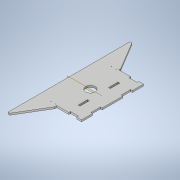
# Autodesk Inventor part: Side_two
Saved by Autodesk Inventor 2020 (Build 240168000, 168)
## iProperties
Created: 2019-12-17
Part Number: Side_two
Material: Generic
Document SubType Name: Modeling
Designer: fabfarm
Density: 1 g/cm^3
Appearance: Default
Author: fabfarm
Autodesk Inventor part; units mm, degrees
ref_plane "YZ Plane" through (0, 0, 0) normal (1, 0, 0) x (0, 1, 0)
ref_plane "XZ Plane" through (0, 0, 0) normal (0, 1, 0) x (-1, 0, 0)
ref_plane "XY Plane" through (0, 0, 0) normal (0, 0, 1) x (1, 0, 0)
sketch "Sketch1" plane through (0, 0, 0) normal (0, 1, 0) x (-1, 0, 0)
  line L0 (0, 0) -> (462.95, 0)
  line L1 (462.95, 0) -> (462.95, 660)
  line L2 (462.95, 660) -> (0, 660)
  line L3 (0, 660) -> (0, 0)
  dimension "d0" = 462.95
  dimension "d1" = 660
  constraints: 8 end point, 2 parallel, 1 horizontal, 1 perpendicular
  measures "d0" distance of L0.start L0.end
  measures "d1" distance of L2.end L0.start
extrude "Extrusion1" add sketch "Sketch1" along normal blind 18.55
ref_plane "Work Plane1" through (-462.95, 0, 330) normal (0, 0, 1) x (1, 0, 0)
sketch "Sketch4" plane through (0, 18.55, 0) normal (0, 1, 0) x (1, 0, 0)
  circle A0 centre (-235, -330) radius 50
  line L0 (92.59, -330) -> (-555.54, -330) projected
  line L1 (0, -660) -> (0, 0) projected
  point P0 (0, -641.45)
  point P1 (0, -18.55)
  dimension "d20" = 100
  dimension "d21" = 235
  constraints: 1 centre point, 1 point on line
  measures "d20" diameter of A0
  measures "d21" distance from line of L1 A0.centre
extrude "Extrusion4" cut sketch "Sketch4" against normal blind 20
sketch "Esquisse5" plane through (0, 18.55, 0) normal (0, 1, 0) x (1, 0, 0)
  line L0 (-462.95, -660) -> (0, -660) projected
  line L1 (-360.1, -660) -> (-259.9, -660)
  line L2 (-259.9, -660) -> (-259.9, -641.45)
  line L3 (-259.9, -641.45) -> (-360.1, -641.45)
  line L4 (-360.1, -641.45) -> (-360.1, -660)
  line L5 (0, 0) -> (-462.95, 0) projected
  line L6 (-360.1, 0) -> (-259.9, 0)
  line L7 (-259.9, 0) -> (-259.9, -18.55)
  line L8 (-259.9, -18.55) -> (-360.1, -18.55)
  line L9 (-360.1, -18.55) -> (-360.1, 0)
  line L10 (-462.95, 0) -> (-462.95, -660) projected
  line L11 (0, -660) -> (0, 0) projected
  point P0 (-463.9, -660)
  point P1 (-463.9, 0)
  point P2 (-259.9, -660)
  dimension "d24" = 100.2
  dimension "d25" = 102.85
  dimension "d26" = 18.55
  dimension "d27" = 18.55
  dimension "d28" = 259.9
  constraints: 16 end point, 4 parallel, 4 point on line, 2 horizontal, 2 perpendicular, 1 other
  measures "d24" distance of L2.end L3.end
  measures "d26" distance of L1.end L2.end
  measures "d27" distance of L6.end L7.end
  measures "d28" distance from line of L11 L1.end
extrude "Extrusion5" [suppressed]
sketch "Esquisse6" plane through (0, 18.55, 0) normal (0, 1, 0) x (1, 0, 0)
  circle A0 centre (-333.95, -7.5) radius 2.25
  circle A1 centre (-283.95, -7.5) radius 2.25
  circle A2 centre (-333.95, -652.5) radius 2.25
  circle A3 centre (-283.95, -652.5) radius 2.25
  line L0 (-462.95, -660) -> (0, -660) projected
  line L1 (0, 0) -> (-462.95, 0) projected
  line L2 (-462.95, 0) -> (-462.95, -660) projected
  dimension "d31" = 4.5
  dimension "d72" = 7.5
  dimension "d73" = 50
  dimension "d75" = 7.5
  dimension "d77" = 129
  dimension "d80" = 50
  dimension "d81" = 129
  constraints: 4 centre point, 3 equal radius, 2 vertical alignment, 1 coincident, 1 horizontal alignment
  measures "d31" diameter of A3
  measures "d72" distance from line of L0 A2.centre
  measures "d73" distance of point (-283.95, -652.5) A2.centre
  measures "d75" distance from line of L1 A0.centre
  measures "d77" distance from line of L2 A0.centre
  measures "d80" distance of A1.centre A0.centre
  measures "d81" distance from line of L2 A2.centre
extrude "Extrusion6" cut sketch "Esquisse6" against normal blind 100
sketch "Esquisse7" plane through (0, 18.55, 0) normal (0, 1, 0) x (1, 0, 0)
  line L0 (-134.85, -541.5) -> (-153.5, -541.5)
  line L1 (-153.5, -541.5) -> (-153.5, -441.4)
  line L2 (-153.5, -441.4) -> (-134.85, -441.4)
  line L3 (-134.85, -441.4) -> (-134.85, -541.5)
  line L4 (-134.85, -218.6) -> (-153.5, -218.6)
  line L5 (-153.5, -218.6) -> (-153.5, -118.5)
  line L6 (-153.5, -118.5) -> (-134.85, -118.5)
  line L7 (-134.85, -118.5) -> (-134.85, -218.6)
  line L8 (0, 0) -> (-462.95, 0) projected
  line L9 (-462.95, -660) -> (0, -660) projected
  line L10 (0, -660) -> (0, 0) projected
  point P0 (-259.9, 0)
  point P1 (-360.1, -660)
  dimension "d34" = 118.5
  dimension "d35" = 100.1
  dimension "d36" = 100.1
  dimension "d37" = 118.5
  dimension "d38" = 18.65
  dimension "d78" = 134.85
  constraints: 16 end point, 4 parallel, 2 collinear, 2 horizontal, 2 perpendicular
  measures "d34" distance between parallel lines of L8 L6
  measures "d35" distance of L4.end L5.end
  measures "d36" distance of L0.end L1.end
  measures "d37" distance between parallel lines of L9 L0
  measures "d38" distance of L1.end L2.end
  measures "d78" distance between parallel lines of L10 L3
extrude "Extrusion7" cut sketch "Esquisse7" against normal blind 20
sketch "Esquisse8" plane through (0, 18.55, 0) normal (0, 1, 0) x (1, 0, 0)
  circle A0 centre (-152.3686, -540.3686) radius 1.6
  circle A1 centre (-152.3686, -442.5314) radius 1.6
  circle A2 centre (-152.3686, -217.4686) radius 1.6
  circle A3 centre (-152.3686, -119.6314) radius 1.6
  line L0 (-152.3686, -119.6314) -> (-153.5, -118.5) construction
  line L1 (-153.5, -118.5) -> (-134.85, -118.5) projected
  point P0 (0, 0)
  point P1 (-153.5, -218.6)
  point P2 (-153.5, -441.4)
  point P3 (-153.5, -541.5)
  dimension "d41" = 3.2
  dimension "d64" = 45
  constraints: 3 vertical alignment, 2 end point, 12 other
  measures "d64" angle of L1 L0
extrude "Extrusion8" cut sketch "Esquisse8" against normal blind 20
sketch "Esquisse9" plane through (0, 18.55, 0) normal (0, 1, 0) x (1, 0, 0)
  line L0 (-135, -660) -> (-135, -641.45)
  line L1 (-135, -641.45) -> (-50, -641.45)
  line L2 (-50, -641.45) -> (-50, -660)
  line L3 (0, -660) -> (0, 0) projected
  line L4 (-50, -660) -> (-135, -660)
  line L5 (-462.95, -660) -> (0, -660) projected
  line L6 (-50, 0) -> (-135, 0)
  line L7 (-135, 0) -> (-135, -18.55)
  line L8 (-135, -18.55) -> (-50, -18.55)
  line L9 (-50, -18.55) -> (-50, 0)
  line L10 (0, 0) -> (-462.95, 0) projected
  point P0 (0, -18.55)
  point P1 (-259.9, -660)
  point P2 (-259.9, 0)
  point P3 (-360.1, -660)
  dimension "d57" = 50
  dimension "d58" = 135
  dimension "d60" = 18.55
  constraints: 16 end point, 5 collinear, 2 horizontal, 2 parallel, 1 perpendicular
  measures "d57" distance between parallel lines of L3 L2
  measures "d58" distance between parallel lines of L3 L0
  measures "d60" distance of L1.end L2.end
extrude "Extrusion9" cut sketch "Esquisse9" against normal blind 20
sketch "Esquisse10" plane through (0, 18.55, 0) normal (0, 1, 0) x (1, 0, 0)
  line L0 (0, -660) -> (0, 0) projected
  line L1 (0, -541.5) -> (-18.55, -541.5)
  line L2 (-18.55, -541.5) -> (-18.55, -441.4)
  line L3 (-18.55, -441.4) -> (0, -441.4)
  line L4 (0, -441.4) -> (0, -541.5)
  line L5 (0, -218.6) -> (-18.55, -218.6)
  line L6 (-18.55, -218.6) -> (-18.55, -118.5)
  line L7 (-18.55, -118.5) -> (0, -118.5)
  line L8 (0, -118.5) -> (0, -218.6)
  line L9 (-134.85, -541.5) -> (-151.2373, -541.5) projected
  line L10 (-151.2373, -441.4) -> (-134.85, -441.4) projected
  line L11 (-134.85, -218.6) -> (-151.2373, -218.6) projected
  line L12 (-151.2373, -118.5) -> (-134.85, -118.5) projected
  point P0 (0, -641.45)
  point P1 (0, -18.55)
  point P2 (0, -441.4)
  point P3 (0, -118.5)
  dimension "d50" = 18.55
  constraints: 16 end point, 4 collinear, 4 parallel, 3 point on line, 2 horizontal, 2 perpendicular
  measures "d50" distance of L1.start L1.end
extrude "Extrusion10" cut sketch "Esquisse10" against normal blind 20
sketch "Esquisse11" plane through (0, 18.55, 0) normal (0, 1, 0) x (1, 0, 0)
  circle A0 centre (-135.9814, -217.4686) radius 1.6
  circle A1 centre (-17.4186, -217.4686) radius 1.6
  circle A2 centre (-135.9814, -119.6314) radius 1.6
  circle A3 centre (-17.4186, -119.6314) radius 1.6
  circle A4 centre (-133.8686, -17.4186) radius 1.6
  line L0 (-50, -18.55) -> (-135, -18.55) projected
  line L1 (-135, -18.55) -> (-133.8686, -17.4186) construction
  line L2 (-135.9814, -119.6314) -> (-134.85, -118.5) construction
  line L3 (-134.85, -118.5) -> (-134.85, -218.6) projected
  circle A5 centre (-51.1314, -17.4186) radius 1.6
  line L4 (0, -441.4) -> (0, -218.6) projected
  line L5 (0, -330) -> (-185, -330) construction
  circle A6 centre (-235, -330) radius 50 construction
  circle A7 centre (-135.9814, -442.5314) radius 1.6
  circle A8 centre (-17.4186, -442.5314) radius 1.6
  circle A9 centre (-135.9814, -540.3686) radius 1.6
  circle A10 centre (-17.4186, -540.3686) radius 1.6
  circle A11 centre (-133.8686, -642.5814) radius 1.6
  line L6 (-135, -641.45) -> (-133.8686, -642.5814) construction
  line L7 (-135.9814, -540.3686) -> (-134.85, -541.5) construction
  circle A12 centre (-51.1314, -642.5814) radius 1.6
  point P0 (0, 0)
  point P1 (-18.55, -541.5)
  point P2 (-18.55, -441.4)
  point P3 (-135, -641.45)
  point P4 (-18.55, -118.5)
  point P5 (-18.55, -218.6)
  point P6 (-18.55, -541.5)
  point P7 (-134.85, -441.4)
  point P8 (-18.55, -441.4)
  point P9 (-52.2627, -18.55)
  dimension "d63" = 3.2
  dimension "d61" = 45
  dimension "d62" = 45
  constraints: 11 symmetric about line, 10 end point, 5 horizontal, 4 horizontal alignment, 3 centre point, 2 vertical alignment, 1 midpoint, 31 other
  measures "d61" angle of L0 L1
  measures "d62" angle of L3 L2
extrude "Extrusion11" cut sketch "Esquisse11" against normal blind 20 contours L3 A0 | A0 L3 | A1 | A2 L3 | L3 A2 | A3 | A4 L0 | L0 A4 | L0 A5 | A7 | A8 | A9 | A10 | A11 | A12 picked at (-51.5143, -17.5621)
sketch "Esquisse12" plane through (0, 18.55, 0) normal (0, 1, 0) x (1, 0, 0)
  line L0 (-462.95, -660) -> (0, -660) projected
  line L1 (-262.95, -660) -> (-262.95, -680)
  line L2 (-262.95, -680) -> (-442.95, -980)
  line L3 (-442.95, -980) -> (-462.95, -980)
  line L4 (-462.95, -980) -> (-462.95, -660)
  circle A0 centre (-235, -330) radius 50 projected
  line L5 (-285, -330) -> (-462.95, -330) construction
  line L6 (-462.95, -660) -> (-262.95, -660)
  line L7 (-462.95, 0) -> (-360.1, 0)
  line L8 (-262.95, 0) -> (-262.95, 20)
  line L9 (-262.95, 20) -> (-442.95, 320)
  line L10 (-442.95, 320) -> (-462.95, 320)
  line L11 (-462.95, 320) -> (-462.95, 0)
  line L12 (-462.95, 0) -> (-262.95, 0)
  line L13 (-462.95, 0) -> (-462.95, -660) projected
  point P0 (0, 0)
  point P1 (-331.7, -652.5)
  dimension "d65" = 320
  dimension "d66" = 20
  dimension "d67" = 20
  dimension "d79" = 200
  constraints: 24 end point, 5 symmetric about line, 2 perpendicular, 2 point on line, 1 collinear, 1 horizontal, 1 horizontal alignment, 1 midpoint, 1 vertical, 1 other
  measures "d65" distance of L3.end L0.start
  measures "d66" distance of L2.end L3.end
  measures "d67" distance of L1.start L1.end
  measures "d79" distance of L0.start L1.start
extrude "Extrusion12" add sketch "Esquisse12" against normal blind 18.55 contours L0 L1 L2 L3 L4 | L11 L10 L9 L8 L12 L7
body "Solid1"
